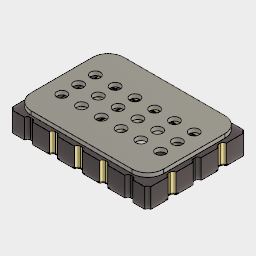
mics-6814_three_gas_sensor.7066ebe4-298e-4c48-8aa3-1ca8056fe42b (Autodesk Fusion 360 design; units mm, degrees)
Autodesk Fusion 360 part; units mm, degrees
sketch "Sketch1" plane through (0, 0, 0) normal (0, 0, 1) x (1, 0, 0) in component "body"
  line L0 (-3.5, 2.5) -> (3.5, 2.5)
  line L1 (3.5, 2.5) -> (3.5, -2.5)
  line L2 (3.5, -2.5) -> (-3.5, -2.5)
  line L3 (-3.5, -2.5) -> (-3.5, 2.5)
  arc A0 (3.35, 2.5) -> (3.5, 2.35) centre (3.5, 2.5) ccw
  arc A1 (3.5, -2.35) -> (3.35, -2.5) centre (3.5, -2.5) ccw
  arc A2 (-3.5, 2.35) -> (-3.35, 2.5) centre (-3.5, 2.5) ccw
  arc A3 (-3.35, -2.5) -> (-3.5, -2.35) centre (-3.5, -2.5) ccw
  line L4 (-0.3, 2.5) -> (0.3, 2.5)
  line L5 (0.3, 2.5) -> (0.3, 1.5)
  line L6 (0.3, 1.5) -> (-0.3, 1.5)
  line L7 (-0.3, 1.5) -> (-0.3, 2.5)
  line L8 (-0.05, 2.35) -> (0.05, 2.35)
  arc A4 (0.05, 2.35) -> (0.2, 2.5) centre (0.05, 2.5) ccw
  arc A5 (-0.2, 2.5) -> (-0.05, 2.35) centre (-0.05, 2.5) ccw
  arc A6 (-2.74, 2.5) -> (-2.59, 2.35) centre (-2.59, 2.5) ccw
  line L9 (-2.59, 2.35) -> (-2.49, 2.35)
  arc A7 (-2.49, 2.35) -> (-2.34, 2.5) centre (-2.49, 2.5) ccw
  arc A8 (-1.47, 2.5) -> (-1.32, 2.35) centre (-1.32, 2.5) ccw
  line L10 (-1.32, 2.35) -> (-1.22, 2.35)
  arc A9 (-1.22, 2.35) -> (-1.07, 2.5) centre (-1.22, 2.5) ccw
  arc A10 (1.07, 2.5) -> (1.22, 2.35) centre (1.22, 2.5) ccw
  line L11 (1.22, 2.35) -> (1.32, 2.35)
  arc A11 (1.32, 2.35) -> (1.47, 2.5) centre (1.32, 2.5) ccw
  arc A12 (2.34, 2.5) -> (2.49, 2.35) centre (2.49, 2.5) ccw
  line L12 (2.49, 2.35) -> (2.59, 2.35)
  arc A13 (2.59, 2.35) -> (2.74, 2.5) centre (2.59, 2.5) ccw
  line L13 (-3.5, 0) -> (3.5, 0) construction
  line L14 (3.35, 0.05) -> (3.35, -0.05)
  arc A14 (3.35, -0.05) -> (3.5, -0.2) centre (3.5, -0.05) ccw
  arc A15 (3.5, 0.2) -> (3.35, 0.05) centre (3.5, 0.05) ccw
  line L15 (-0.05, -2.35) -> (0.05, -2.35)
  arc A16 (0.2, -2.5) -> (0.05, -2.35) centre (0.05, -2.5) ccw
  arc A17 (-0.05, -2.35) -> (-0.2, -2.5) centre (-0.05, -2.5) ccw
  arc A18 (-2.59, -2.35) -> (-2.74, -2.5) centre (-2.59, -2.5) ccw
  line L16 (-2.59, -2.35) -> (-2.49, -2.35)
  arc A19 (-2.34, -2.5) -> (-2.49, -2.35) centre (-2.49, -2.5) ccw
  arc A20 (-1.32, -2.35) -> (-1.47, -2.5) centre (-1.32, -2.5) ccw
  line L17 (-1.32, -2.35) -> (-1.22, -2.35)
  arc A21 (-1.07, -2.5) -> (-1.22, -2.35) centre (-1.22, -2.5) ccw
  arc A22 (1.22, -2.35) -> (1.07, -2.5) centre (1.22, -2.5) ccw
  line L18 (1.22, -2.35) -> (1.32, -2.35)
  arc A23 (1.47, -2.5) -> (1.32, -2.35) centre (1.32, -2.5) ccw
  arc A24 (2.49, -2.35) -> (2.34, -2.5) centre (2.49, -2.5) ccw
  line L19 (2.49, -2.35) -> (2.59, -2.35)
  arc A25 (2.74, -2.5) -> (2.59, -2.35) centre (2.59, -2.5) ccw
  arc A26 (3.5, -1.07) -> (3.35, -1.22) centre (3.5, -1.22) ccw
  line L20 (3.35, -1.22) -> (3.35, -1.32)
  arc A27 (3.35, -1.32) -> (3.5, -1.47) centre (3.5, -1.32) ccw
  arc A28 (3.5, 1.47) -> (3.35, 1.32) centre (3.5, 1.32) ccw
  line L21 (3.35, 1.32) -> (3.35, 1.22)
  arc A29 (3.35, 1.22) -> (3.5, 1.07) centre (3.5, 1.22) ccw
  line L22 (-3.35, 0.05) -> (-3.35, -0.05)
  arc A30 (-3.5, -0.2) -> (-3.35, -0.05) centre (-3.5, -0.05) ccw
  arc A31 (-3.35, 0.05) -> (-3.5, 0.2) centre (-3.5, 0.05) ccw
  arc A32 (-3.35, -1.22) -> (-3.5, -1.07) centre (-3.5, -1.22) ccw
  line L23 (-3.35, -1.22) -> (-3.35, -1.32)
  arc A33 (-3.5, -1.47) -> (-3.35, -1.32) centre (-3.5, -1.32) ccw
  arc A34 (-3.35, 1.32) -> (-3.5, 1.47) centre (-3.5, 1.32) ccw
  line L24 (-3.35, 1.32) -> (-3.35, 1.22)
  arc A35 (-3.5, 1.07) -> (-3.35, 1.22) centre (-3.5, 1.22) ccw
  line L25 (-0.97, 2.5) -> (-0.97, 1.5)
  line L26 (-0.97, 1.5) -> (-1.57, 1.5)
  line L27 (-1.57, 1.5) -> (-1.57, 2.5)
  line L28 (1.57, 2.5) -> (1.57, 1.5)
  line L29 (1.57, 1.5) -> (0.97, 1.5)
  line L30 (0.97, 1.5) -> (0.97, 2.5)
  line L31 (-0.3, -2.5) -> (-0.3, -1.5)
  line L32 (-0.3, -1.5) -> (0.3, -1.5)
  line L33 (0.3, -1.5) -> (0.3, -2.5)
  line L34 (-1.57, -2.5) -> (-1.57, -1.5)
  line L35 (-1.57, -1.5) -> (-0.97, -1.5)
  line L36 (-0.97, -1.5) -> (-0.97, -2.5)
  line L37 (0.97, -2.5) -> (0.97, -1.5)
  line L38 (0.97, -1.5) -> (1.57, -1.5)
  line L39 (1.57, -1.5) -> (1.57, -2.5)
  line L40 (3.5, -0.97) -> (2.5, -0.97)
  line L41 (2.5, -0.97) -> (2.5, -1.57)
  line L42 (2.5, -1.57) -> (3.5, -1.57)
  line L43 (3.5, 1.57) -> (2.5, 1.57)
  line L44 (2.5, 1.57) -> (2.5, 0.97)
  line L45 (2.5, 0.97) -> (3.5, 0.97)
  line L46 (-3.5, 1.57) -> (-2.5, 1.57)
  line L47 (-2.5, 1.57) -> (-2.5, 0.97)
  line L48 (-2.5, 0.97) -> (-3.5, 0.97)
  line L49 (-3.5, -0.97) -> (-2.5, -0.97)
  line L50 (-2.5, -0.97) -> (-2.5, -1.57)
  line L51 (-2.5, -1.57) -> (-3.5, -1.57)
  circle A36 centre (1.25, 0.97) radius 0.2
  dimension "d1" = 5
  dimension "d2" = 7
  dimension "d3" = 0.3
  dimension "d4" = 0.3
  dimension "d5" = 0.3
  dimension "d6" = 0.3
  dimension "d8" = 0.6
  dimension "d9" = 1
  dimension "d10" = 0.15
  dimension "d11" = 0.15
  dimension "d12" = 0.15
  dimension "d13" = 0.4
  dimension "d16" = 1.27
  dimension "d17" = 0
  dimension "d18" = 0.15
  dimension "d19" = 0.15
  dimension "d20" = 0.15
  dimension "d21" = 0.4
  dimension "d27" = 0.15
  dimension "d28" = 0.15
  dimension "d29" = 0.4
  dimension "d32" = 1.27
  dimension "d33" = 0
  dimension "d34" = 0.15
  dimension "d37" = 0
  dimension "d38" = 1.27
  dimension "d39" = 0.15
  dimension "d40" = 0.15
  dimension "d41" = 0.15
  dimension "d42" = 0.4
  dimension "d45" = 0
  dimension "d46" = 1.27
  dimension "d49" = 1.27
  dimension "d50" = 0
  dimension "d51" = 1
  dimension "d52" = 0.6
  dimension "d55" = 1.27
  dimension "d56" = 0
  dimension "d57" = 1
  dimension "d58" = 0.6
  dimension "d59" = 1
  dimension "d60" = 0.6
  dimension "d61" = 1
  dimension "d62" = 0.6
  dimension "d63" = 1
  dimension "d64" = 0.6
  dimension "d65" = 0.4
  dimension "d67" = 1.25
  dimension "d92" = 0.97
  constraint horizontal L0
  constraint vertical L1
  constraint horizontal L2
  constraint vertical L3
  constraint coincident L1
  constraint coincident L0
  constraint coincident L2
  constraint coincident L3
  constraint midpoint L3
  constraint midpoint L0
  constraint horizontal L4
  constraint vertical L5
  constraint horizontal L6
  constraint vertical L7
  constraint midpoint L6
  constraint horizontal L8
  constraint coincident L4
  constraint tangent L8 A4
  constraint tangent L8 A5
  constraint midpoint L8
  constraint midpoint L1
  constraint tangent L14 A14
  constraint tangent L14 A15
  constraint vertical L14
  constraint tangent L15 A16
  constraint tangent L15 A17
  constraint horizontal L15
  constraint midpoint L15
  constraint tangent L22 A30
  constraint tangent L22 A31
  constraint vertical L22
  constraint midpoint L22
  constraint horizontal L32
  constraint vertical L31
  constraint vertical L33
  constraint midpoint L32
  constraint vertical L41
  constraint horizontal L40
  constraint horizontal L42
  constraint midpoint L41
  constraint midpoint L20
  constraint midpoint L44
  constraint midpoint L21
  constraint vertical L44
  constraint horizontal L43
  constraint horizontal L45
  constraint midpoint L47
  constraint midpoint L24
  constraint horizontal L46
  constraint horizontal L48
  constraint vertical L47
  constraint midpoint L50
  constraint midpoint L23
  constraint horizontal L49
  constraint horizontal L51
  constraint vertical L50
  constraint midpoint L14
  measures "d2" distance of L1 L3
  measures "d3" diameter of A2
  measures "d4" diameter of A3
  measures "d5" diameter of A1
  measures "d6" diameter of A0
  measures "d10" distance of L0 L8
  measures "d11" radius of A4
  measures "d12" radius of A5
  measures "d18" distance of L1 L14
  measures "d19" radius of A14
  measures "d20" radius of A15
  measures "d27" radius of A16
  measures "d28" radius of A17
  measures "d34" distance of L2
  measures "d39" distance of L3 L22
  measures "d40" radius of A31
  measures "d41" radius of A30
  measures "d51" distance of L2 L32
  measures "d52" distance of L31 L33
  measures "d57" distance of L1 L41
  measures "d58" distance of L40 L42
  measures "d59" distance of L1 L44
  measures "d60" distance of L43 L45
  measures "d61" distance of L3 L47
  measures "d62" distance of L46 L48
  measures "d63" distance of L3 L50
  measures "d64" distance of L49 L51
  measures "d65" diameter of A36
extrude "Extrude1" add sketch "Sketch1" along normal blind 1 contours L0 L1 L2 L3 A0 A1 A2 A3 L5 L6 L7 A6 L9 A7 A12 L12 A13 L14 A14 A15 A18 L16 A19 A24 L19 A25 L22 A30 A31 L25 L26 L27 L28 L29 L30 L31 L32 L33 L34 L35 L36 L37 L38 L39 L40 L41 L42 L43 L44 L45 L46 L47 L48 L49 L50 L51 | L3 A34 L24 A35 L46 L47 L48 | L0 A8 L10 A9 L25 L26 L27 | L0 L4 L5 L6 L7 L8 A4 A5 | L3 A32 L23 A33 L49 L50 L51 | L0 A10 L11 A11 L28 L29 L30 | L2 A20 L17 A21 L34 L35 L36 | L1 A28 L21 A29 L43 L44 L45 | L2 L15 A16 A17 L31 L32 L33 | L2 A22 L18 A23 L37 L38 L39 | L1 A26 L20 A27 L40 L41 L42 | A36 makes body 1 in component "body"
extrude "Extrude2" add sketch "Sketch1" along normal blind 0.05 separate body contours L3 A34 L24 A35 L46 L47 L48 | L0 A8 L10 A9 L25 L26 L27 | L0 L4 L5 L6 L7 L8 A4 A5 | L3 A32 L23 A33 L49 L50 L51 | L0 A10 L11 A11 L28 L29 L30 | L2 A20 L17 A21 L34 L35 L36 | L1 A28 L21 A29 L43 L44 L45 | L2 L15 A16 A17 L31 L32 L33 | L2 A22 L18 A23 L37 L38 L39 | L1 A26 L20 A27 L40 L41 L42 | A36 makes body 2 at (-0.0167, -1.7833, 0) makes body 3 at (-1.2533, 1.7833, 0) makes body 4 at (2.7833, -1.2867, 0) makes body 5 at (0.0167, 1.7833, 0) makes body 6 at (-1.2867, -1.7833, 0) makes body 7 at (1.2867, -1.7833, 0) makes body 8 at (-2.7833, 1.2533, 0) makes body 9 at (2.7833, 1.2867, 0) makes body 10 at (1.2867, 1.7833, 0) makes body 11 at (-2.7833, -1.2533, 0) makes body 12 at (1.4078, 0.9411, 0) in component "body"
combine "Combine1" operation cut target body 1 tool bodies 7 2 6 11 8 3 5 10 12 4 9 keep tools in component "body"
sketch "Sketch1 (2)" plane through (0, 0, 1) normal (0, 0, 1) x (-1, 0, 0) in component "lid"
  line L0 (3.35, -0.05) -> (3.35, 0.05)
  arc A0 (3.5, 0.2) -> (3.35, 0.05) centre (3.5, 0.05) ccw
  line L1 (3.5, 0.2) -> (3.5, 1.07)
  arc A1 (3.35, 1.22) -> (3.5, 1.07) centre (3.5, 1.22) ccw
  line L2 (3.35, 1.22) -> (3.35, 1.32)
  arc A2 (3.5, 1.47) -> (3.35, 1.32) centre (3.5, 1.32) ccw
  line L3 (3.5, 1.47) -> (3.5, 2.35)
  arc A3 (3.35, 2.5) -> (3.5, 2.35) centre (3.5, 2.5) ccw
  line L4 (3.35, 2.5) -> (2.74, 2.5)
  arc A4 (2.59, 2.35) -> (2.74, 2.5) centre (2.59, 2.5) ccw
  line L5 (2.59, 2.35) -> (2.49, 2.35)
  arc A5 (2.34, 2.5) -> (2.49, 2.35) centre (2.49, 2.5) ccw
  line L6 (2.34, 2.5) -> (1.47, 2.5)
  arc A6 (1.32, 2.35) -> (1.47, 2.5) centre (1.32, 2.5) ccw
  line L7 (1.32, 2.35) -> (1.22, 2.35)
  arc A7 (1.07, 2.5) -> (1.22, 2.35) centre (1.22, 2.5) ccw
  line L8 (1.07, 2.5) -> (0.2, 2.5)
  arc A8 (0.05, 2.35) -> (0.2, 2.5) centre (0.05, 2.5) ccw
  line L9 (0.05, 2.35) -> (-0.05, 2.35)
  arc A9 (-0.2, 2.5) -> (-0.05, 2.35) centre (-0.05, 2.5) ccw
  line L10 (-0.2, 2.5) -> (-1.07, 2.5)
  arc A10 (-1.22, 2.35) -> (-1.07, 2.5) centre (-1.22, 2.5) ccw
  line L11 (-1.22, 2.35) -> (-1.32, 2.35)
  arc A11 (-1.47, 2.5) -> (-1.32, 2.35) centre (-1.32, 2.5) ccw
  line L12 (-1.47, 2.5) -> (-2.34, 2.5)
  arc A12 (-2.49, 2.35) -> (-2.34, 2.5) centre (-2.49, 2.5) ccw
  line L13 (-2.49, 2.35) -> (-2.59, 2.35)
  arc A13 (-2.74, 2.5) -> (-2.59, 2.35) centre (-2.59, 2.5) ccw
  line L14 (-2.74, 2.5) -> (-3.35, 2.5)
  arc A14 (-3.5, 2.35) -> (-3.35, 2.5) centre (-3.5, 2.5) ccw
  line L15 (-3.5, 2.35) -> (-3.5, 1.47)
  arc A15 (-3.35, 1.32) -> (-3.5, 1.47) centre (-3.5, 1.32) ccw
  line L16 (-3.35, 1.32) -> (-3.35, 1.22)
  arc A16 (-3.5, 1.07) -> (-3.35, 1.22) centre (-3.5, 1.22) ccw
  line L17 (-3.5, 1.07) -> (-3.5, 0.2)
  arc A17 (-3.35, 0.05) -> (-3.5, 0.2) centre (-3.5, 0.05) ccw
  line L18 (-3.35, 0.05) -> (-3.35, -0.05)
  arc A18 (-3.5, -0.2) -> (-3.35, -0.05) centre (-3.5, -0.05) ccw
  line L19 (-3.5, -0.2) -> (-3.5, -1.07)
  arc A19 (-3.35, -1.22) -> (-3.5, -1.07) centre (-3.5, -1.22) ccw
  line L20 (-3.35, -1.22) -> (-3.35, -1.32)
  arc A20 (-3.5, -1.47) -> (-3.35, -1.32) centre (-3.5, -1.32) ccw
  line L21 (-3.5, -1.47) -> (-3.5, -2.35)
  arc A21 (-3.35, -2.5) -> (-3.5, -2.35) centre (-3.5, -2.5) ccw
  line L22 (-3.35, -2.5) -> (-2.74, -2.5)
  arc A22 (-2.59, -2.35) -> (-2.74, -2.5) centre (-2.59, -2.5) ccw
  line L23 (-2.59, -2.35) -> (-2.49, -2.35)
  arc A23 (-2.34, -2.5) -> (-2.49, -2.35) centre (-2.49, -2.5) ccw
  line L24 (-2.34, -2.5) -> (-1.47, -2.5)
  arc A24 (-1.32, -2.35) -> (-1.47, -2.5) centre (-1.32, -2.5) ccw
  line L25 (-1.32, -2.35) -> (-1.22, -2.35)
  arc A25 (-1.07, -2.5) -> (-1.22, -2.35) centre (-1.22, -2.5) ccw
  line L26 (-1.07, -2.5) -> (-0.2, -2.5)
  arc A26 (-0.05, -2.35) -> (-0.2, -2.5) centre (-0.05, -2.5) ccw
  line L27 (-0.05, -2.35) -> (0.05, -2.35)
  arc A27 (0.2, -2.5) -> (0.05, -2.35) centre (0.05, -2.5) ccw
  line L28 (0.2, -2.5) -> (1.07, -2.5)
  arc A28 (1.22, -2.35) -> (1.07, -2.5) centre (1.22, -2.5) ccw
  line L29 (1.22, -2.35) -> (1.32, -2.35)
  arc A29 (1.47, -2.5) -> (1.32, -2.35) centre (1.32, -2.5) ccw
  line L30 (1.47, -2.5) -> (2.34, -2.5)
  arc A30 (2.49, -2.35) -> (2.34, -2.5) centre (2.49, -2.5) ccw
  line L31 (2.49, -2.35) -> (2.59, -2.35)
  arc A31 (2.74, -2.5) -> (2.59, -2.35) centre (2.59, -2.5) ccw
  line L32 (2.74, -2.5) -> (3.35, -2.5)
  arc A32 (3.5, -2.35) -> (3.35, -2.5) centre (3.5, -2.5) ccw
  line L33 (3.5, -2.35) -> (3.5, -1.47)
  arc A33 (3.35, -1.32) -> (3.5, -1.47) centre (3.5, -1.32) ccw
  line L34 (3.35, -1.32) -> (3.35, -1.22)
  arc A34 (3.5, -1.07) -> (3.35, -1.22) centre (3.5, -1.22) ccw
  line L35 (3.5, -1.07) -> (3.5, -0.2)
  arc A35 (3.35, -0.05) -> (3.5, -0.2) centre (3.5, -0.05) ccw
  line L36 (2.55, -2.35) -> (-2.55, -2.35)
  line L37 (-3.35, -1.55) -> (-3.35, 1.55)
  line L38 (-2.55, 2.35) -> (2.55, 2.35)
  line L39 (3.35, 1.55) -> (3.35, -1.55)
  arc A36 (2.55, -2.35) -> (3.35, -1.55) centre (2.55, -1.55) ccw
  arc A37 (3.35, 1.55) -> (2.55, 2.35) centre (2.55, 1.55) ccw
  arc A38 (-3.35, -1.55) -> (-2.55, -2.35) centre (-2.55, -1.55) ccw
  arc A39 (-2.55, 2.35) -> (-3.35, 1.55) centre (-2.55, 1.55) ccw
  circle A40 centre (2.5, 0) radius 0.25
  circle A41 centre (2.5, -0.85) radius 0.25
  circle A42 centre (1.5, -0.85) radius 0.25
  circle A43 centre (0.5, -0.85) radius 0.25
  circle A44 centre (-0.5, -0.85) radius 0.25
  circle A45 centre (-1.5, -0.85) radius 0.25
  circle A46 centre (-2.5, -0.85) radius 0.25
  circle A47 centre (1.5, 0) radius 0.25
  circle A48 centre (0.5, 0) radius 0.25
  circle A49 centre (-0.5, 0) radius 0.25
  circle A50 centre (-1.5, 0) radius 0.25
  circle A51 centre (-2.5, 0) radius 0.25
  circle A52 centre (2.5, 0.85) radius 0.25
  circle A53 centre (1.5, 0.85) radius 0.25
  circle A54 centre (0.5, 0.85) radius 0.25
  circle A55 centre (-0.5, 0.85) radius 0.25
  circle A56 centre (-1.5, 0.85) radius 0.25
  circle A57 centre (-2.5, 0.85) radius 0.25
  dimension "d72" = 4.7
  dimension "d73" = 6.7
  dimension "d74" = 0.8
  dimension "d75" = 0.5
  dimension "d76" = 2.5
  dimension "d79" = -5
  dimension "d80" = 0.85
  constraint horizontal L36
  constraint vertical L37
  constraint horizontal L38
  constraint vertical L39
  constraint midpoint L36
  constraint midpoint L37
  constraint tangent L36 A36
  constraint tangent L39 A36
  constraint tangent L38 A37
  constraint tangent L39 A37
  constraint equal A36 A37
  constraint tangent L36 A38
  constraint tangent L37 A38
  constraint equal A36 A38
  constraint tangent L37 A39
  constraint tangent L38 A39
  constraint equal A36 A39
  measures "d72" distance of L36 L38
  measures "d73" distance of L37 L39
  measures "d74" radius of A36
  measures "d75" diameter of A40
extrude "Extrude1'" add sketch "Sketch1 (2)" along normal blind 0.2 separate body contours L0 L2 L5 L7 L9 L11 L13 L16 L18 L20 L23 L25 L27 L29 L31 L34 L36 L37 L38 L39 A36 A37 A38 A39 makes body 13 in component "lid"
move_body "MoveBody1" bodies 13 to x (1, 0, 0) y (0, 1, 0) z (0, 0, 1) at (0, 0, 0.1) in component "lid"
sketch "Sketch1 (1)" plane through (0, 0, 1) normal (0, 0, 1) x (-1, 0, 0) in component "body"
  line L0 (3.35, -0.05) -> (3.35, 0.05)
  arc A0 (3.5, 0.2) -> (3.35, 0.05) centre (3.5, 0.05) ccw
  line L1 (3.5, 0.2) -> (3.5, 1.07)
  arc A1 (3.35, 1.22) -> (3.5, 1.07) centre (3.5, 1.22) ccw
  line L2 (3.35, 1.22) -> (3.35, 1.32)
  arc A2 (3.5, 1.47) -> (3.35, 1.32) centre (3.5, 1.32) ccw
  line L3 (3.5, 1.47) -> (3.5, 2.35)
  arc A3 (3.35, 2.5) -> (3.5, 2.35) centre (3.5, 2.5) ccw
  line L4 (3.35, 2.5) -> (2.74, 2.5)
  arc A4 (2.59, 2.35) -> (2.74, 2.5) centre (2.59, 2.5) ccw
  line L5 (2.59, 2.35) -> (2.49, 2.35)
  arc A5 (2.34, 2.5) -> (2.49, 2.35) centre (2.49, 2.5) ccw
  line L6 (2.34, 2.5) -> (1.47, 2.5)
  arc A6 (1.32, 2.35) -> (1.47, 2.5) centre (1.32, 2.5) ccw
  line L7 (1.32, 2.35) -> (1.22, 2.35)
  arc A7 (1.07, 2.5) -> (1.22, 2.35) centre (1.22, 2.5) ccw
  line L8 (1.07, 2.5) -> (0.2, 2.5)
  arc A8 (0.05, 2.35) -> (0.2, 2.5) centre (0.05, 2.5) ccw
  line L9 (0.05, 2.35) -> (-0.05, 2.35)
  arc A9 (-0.2, 2.5) -> (-0.05, 2.35) centre (-0.05, 2.5) ccw
  line L10 (-0.2, 2.5) -> (-1.07, 2.5)
  arc A10 (-1.22, 2.35) -> (-1.07, 2.5) centre (-1.22, 2.5) ccw
  line L11 (-1.22, 2.35) -> (-1.32, 2.35)
  arc A11 (-1.47, 2.5) -> (-1.32, 2.35) centre (-1.32, 2.5) ccw
  line L12 (-1.47, 2.5) -> (-2.34, 2.5)
  arc A12 (-2.49, 2.35) -> (-2.34, 2.5) centre (-2.49, 2.5) ccw
  line L13 (-2.49, 2.35) -> (-2.59, 2.35)
  arc A13 (-2.74, 2.5) -> (-2.59, 2.35) centre (-2.59, 2.5) ccw
  line L14 (-2.74, 2.5) -> (-3.35, 2.5)
  arc A14 (-3.5, 2.35) -> (-3.35, 2.5) centre (-3.5, 2.5) ccw
  line L15 (-3.5, 2.35) -> (-3.5, 1.47)
  arc A15 (-3.35, 1.32) -> (-3.5, 1.47) centre (-3.5, 1.32) ccw
  line L16 (-3.35, 1.32) -> (-3.35, 1.22)
  arc A16 (-3.5, 1.07) -> (-3.35, 1.22) centre (-3.5, 1.22) ccw
  line L17 (-3.5, 1.07) -> (-3.5, 0.2)
  arc A17 (-3.35, 0.05) -> (-3.5, 0.2) centre (-3.5, 0.05) ccw
  line L18 (-3.35, 0.05) -> (-3.35, -0.05)
  arc A18 (-3.5, -0.2) -> (-3.35, -0.05) centre (-3.5, -0.05) ccw
  line L19 (-3.5, -0.2) -> (-3.5, -1.07)
  arc A19 (-3.35, -1.22) -> (-3.5, -1.07) centre (-3.5, -1.22) ccw
  line L20 (-3.35, -1.22) -> (-3.35, -1.32)
  arc A20 (-3.5, -1.47) -> (-3.35, -1.32) centre (-3.5, -1.32) ccw
  line L21 (-3.5, -1.47) -> (-3.5, -2.35)
  arc A21 (-3.35, -2.5) -> (-3.5, -2.35) centre (-3.5, -2.5) ccw
  line L22 (-3.35, -2.5) -> (-2.74, -2.5)
  arc A22 (-2.59, -2.35) -> (-2.74, -2.5) centre (-2.59, -2.5) ccw
  line L23 (-2.59, -2.35) -> (-2.49, -2.35)
  arc A23 (-2.34, -2.5) -> (-2.49, -2.35) centre (-2.49, -2.5) ccw
  line L24 (-2.34, -2.5) -> (-1.47, -2.5)
  arc A24 (-1.32, -2.35) -> (-1.47, -2.5) centre (-1.32, -2.5) ccw
  line L25 (-1.32, -2.35) -> (-1.22, -2.35)
  arc A25 (-1.07, -2.5) -> (-1.22, -2.35) centre (-1.22, -2.5) ccw
  line L26 (-1.07, -2.5) -> (-0.2, -2.5)
  arc A26 (-0.05, -2.35) -> (-0.2, -2.5) centre (-0.05, -2.5) ccw
  line L27 (-0.05, -2.35) -> (0.05, -2.35)
  arc A27 (0.2, -2.5) -> (0.05, -2.35) centre (0.05, -2.5) ccw
  line L28 (0.2, -2.5) -> (1.07, -2.5)
  arc A28 (1.22, -2.35) -> (1.07, -2.5) centre (1.22, -2.5) ccw
  line L29 (1.22, -2.35) -> (1.32, -2.35)
  arc A29 (1.47, -2.5) -> (1.32, -2.35) centre (1.32, -2.5) ccw
  line L30 (1.47, -2.5) -> (2.34, -2.5)
  arc A30 (2.49, -2.35) -> (2.34, -2.5) centre (2.49, -2.5) ccw
  line L31 (2.49, -2.35) -> (2.59, -2.35)
  arc A31 (2.74, -2.5) -> (2.59, -2.35) centre (2.59, -2.5) ccw
  line L32 (2.74, -2.5) -> (3.35, -2.5)
  arc A32 (3.5, -2.35) -> (3.35, -2.5) centre (3.5, -2.5) ccw
  line L33 (3.5, -2.35) -> (3.5, -1.47)
  arc A33 (3.35, -1.32) -> (3.5, -1.47) centre (3.5, -1.32) ccw
  line L34 (3.35, -1.32) -> (3.35, -1.22)
  arc A34 (3.5, -1.07) -> (3.35, -1.22) centre (3.5, -1.22) ccw
  line L35 (3.5, -1.07) -> (3.5, -0.2)
  arc A35 (3.35, -0.05) -> (3.5, -0.2) centre (3.5, -0.05) ccw
  line L36 (2.575, -1.875) -> (-2.575, -1.875)
  line L37 (-2.875, -1.575) -> (-2.875, 1.575)
  line L38 (-2.575, 1.875) -> (2.575, 1.875)
  line L39 (2.875, 1.575) -> (2.875, -1.575)
  arc A36 (2.575, -1.875) -> (2.875, -1.575) centre (2.575, -1.575) ccw
  arc A37 (-2.875, -1.575) -> (-2.575, -1.875) centre (-2.575, -1.575) ccw
  arc A38 (-2.575, 1.875) -> (-2.875, 1.575) centre (-2.575, 1.575) ccw
  arc A39 (2.875, 1.575) -> (2.575, 1.875) centre (2.575, 1.575) ccw
  dimension "d83" = 3.75
  dimension "d84" = 5.75
  dimension "d85" = 0.3
  constraint horizontal L36
  constraint vertical L37
  constraint horizontal L38
  constraint vertical L39
  constraint midpoint L37
  constraint midpoint L38
  constraint tangent L36 A36
  constraint tangent L39 A36
  constraint tangent L36 A37
  constraint tangent L37 A37
  constraint equal A36 A37
  constraint tangent L37 A38
  constraint tangent L38 A38
  constraint equal A36 A38
  constraint tangent L38 A39
  constraint tangent L39 A39
  constraint equal A36 A39
  measures "d83" distance of L36 L38
  measures "d84" distance of L37 L39
  measures "d85" radius of A36
extrude "Extrude3" cut sketch "Sketch1 (1)" against normal blind 0.5 contours L36 L37 L38 L39 A36 A37 A38 A39 bodies 1 in component "body"
sketch "Sketch2" plane through (0, 0, 0.5) normal (0, 0, 1) x (-1, 0, 0) in component "body"
  arc A0 (2.575, -1.875) -> (2.875, -1.575) centre (2.575, -1.575) ccw
  line L0 (2.875, -1.575) -> (2.875, 1.575)
  arc A1 (2.875, 1.575) -> (2.575, 1.875) centre (2.575, 1.575) ccw
  line L1 (2.575, 1.875) -> (-2.575, 1.875)
  arc A2 (-2.575, 1.875) -> (-2.875, 1.575) centre (-2.575, 1.575) ccw
  line L2 (-2.875, 1.575) -> (-2.875, -1.575)
  arc A3 (-2.875, -1.575) -> (-2.575, -1.875) centre (-2.575, -1.575) ccw
  line L3 (-2.575, -1.875) -> (2.575, -1.875)
  line L4 (2.75, -1.25) -> (-2.75, -1.25)
  line L5 (-2.75, -1.25) -> (-2.75, 1.25)
  line L6 (-2.75, 1.25) -> (2.75, 1.25)
  line L7 (2.75, 1.25) -> (2.75, -1.25)
  dimension "d88" = 2.5
  dimension "d89" = 5.5
  constraint horizontal L4
  constraint vertical L5
  constraint horizontal L6
  constraint vertical L7
  constraint midpoint L7
  constraint midpoint L4
extrude "Extrude4" add sketch "Sketch2" along normal blind 0.3 bodies 1 in component "body"
sketch "Sketch2 (1)" plane through (0, 0, 0.8) normal (0, 0, 1) x (-1, 0, 0) in component "body"
  line L0 (-2.75, 1.25) -> (2.75, 1.25)
  line L1 (2.75, 1.25) -> (2.75, -1.25)
  line L2 (2.75, -1.25) -> (-2.75, -1.25)
  line L3 (-2.75, -1.25) -> (-2.75, 1.25)
  line L4 (-2.575, -1.875) -> (2.575, -1.875)
  arc A0 (2.575, -1.875) -> (2.875, -1.575) centre (2.575, -1.575) ccw
  line L5 (2.875, -1.575) -> (2.875, 1.575)
  arc A1 (2.875, 1.575) -> (2.575, 1.875) centre (2.575, 1.575) ccw
  line L6 (2.575, 1.875) -> (-2.575, 1.875)
  arc A2 (-2.575, 1.875) -> (-2.875, 1.575) centre (-2.575, 1.575) ccw
  line L7 (-2.875, 1.575) -> (-2.875, -1.575)
  arc A3 (-2.875, -1.575) -> (-2.575, -1.875) centre (-2.575, -1.575) ccw
  arc A4 (2.575, -1.875) -> (2.875, -1.575) centre (2.575, -1.575) ccw
  line L8 (2.875, 1.575) -> (2.875, -1.575)
  line L9 (2.575, -1.875) -> (-2.575, -1.875)
  line L10 (2.75, -1.25) -> (-2.75, -1.25)
  line L11 (-2.75, 1.25) -> (2.75, 1.25)
  arc A5 (2.875, 1.575) -> (2.575, 1.875) centre (2.575, 1.575) ccw
  line L12 (-2.575, 1.875) -> (2.575, 1.875)
  arc A6 (-2.575, 1.875) -> (-2.875, 1.575) centre (-2.575, 1.575) ccw
  line L13 (-2.875, -1.575) -> (-2.875, 1.575)
  arc A7 (-2.875, -1.575) -> (-2.575, -1.875) centre (-2.575, -1.575) ccw
  line L14 (1.375, -1.25) -> (1.375, -1.875)
  line L15 (0.825, -1.25) -> (0.825, -1.875)
  line L16 (0.325, -1.25) -> (0.325, -1.875)
  line L17 (-0.225, -1.25) -> (-0.225, -1.875)
  line L18 (-0.725, -1.25) -> (-0.725, -1.875)
  line L19 (-1.275, -1.25) -> (-1.275, -1.875)
  line L20 (-1.775, -1.25) -> (-1.775, -1.875)
  line L21 (-2.275, -1.25) -> (-2.275, -1.575)
  line L22 (-2.275, -1.575) -> (-2.875, -1.575)
  line L23 (2.375, 1.25) -> (2.375, 1.575)
  line L24 (2.375, 1.575) -> (2.875, 1.575)
  line L25 (1.875, 1.25) -> (1.875, 1.875)
  line L26 (1.375, 1.25) -> (1.375, 1.875)
  line L27 (0.825, 1.25) -> (0.825, 1.875)
  line L28 (0.325, 1.25) -> (0.325, 1.875)
  line L29 (-0.225, 1.25) -> (-0.225, 1.875)
  line L30 (-0.725, 1.25) -> (-0.725, 1.875)
  line L31 (-1.275, 1.25) -> (-1.275, 1.875)
  line L32 (-1.775, 1.25) -> (-1.775, 1.875)
  line L33 (-2.275, 1.25) -> (-2.275, 1.575)
  line L34 (-2.275, 1.575) -> (-2.875, 1.575)
  line L35 (1.875, -1.875) -> (1.875, -1.25)
  line L36 (2.75, -1.25) -> (2.875, -1.25)
  dimension "d95" = 0.55
  dimension "d96" = 0.5
  dimension "d97" = 0.55
  dimension "d98" = 0.5
  dimension "d99" = 0.55
  dimension "d100" = 0.5
  dimension "d101" = 0.5
  dimension "d102" = 1
  dimension "d103" = 0.5
  dimension "d104" = 0.5
  dimension "d105" = 0.55
  dimension "d106" = 0.5
  dimension "d107" = 0.55
  dimension "d108" = 0.5
  dimension "d109" = 0.55
  dimension "d110" = 0.5
  dimension "d111" = 0.5
  dimension "d112" = 1
  dimension "d113" = 0.5
  constraint coincident L10
  constraint coincident L9
  constraint vertical L14
  constraint vertical L15
  constraint vertical L16
  constraint vertical L17
  constraint vertical L18
  constraint vertical L19
  constraint vertical L20
  constraint horizontal L22
  constraint vertical L21
  constraint coincident L11
  constraint horizontal L24
  constraint vertical L23
  constraint coincident L12
  constraint horizontal L34
  constraint vertical L33
  constraint vertical L32
  constraint vertical L31
  constraint vertical L30
  constraint vertical L29
  constraint vertical L28
  constraint vertical L27
  constraint vertical L26
  constraint vertical L25
  constraint vertical L35
  constraint coincident L8
  constraint horizontal L36
  measures "d95" distance of L14 L15
  measures "d96" distance of L15 L16
  measures "d97" distance of L16 L17
  measures "d98" distance of L17 L18
  measures "d99" distance of L18 L19
  measures "d100" distance of L19 L20
  measures "d101" distance of L20 L21
  measures "d102" distance of L8 L25
  measures "d103" distance of L23 L25
  measures "d104" distance of L25 L26
  measures "d105" distance of L26 L27
  measures "d106" distance of L27 L28
  measures "d107" distance of L28 L29
  measures "d108" distance of L29 L30
  measures "d109" distance of L30 L31
  measures "d110" distance of L31 L32
  measures "d111" distance of L32 L33
  measures "d112" distance of L8 L35
  measures "d113" distance of L14 L35
extrude "Extrude5" add sketch "Sketch2 (1)" against normal blind 0.05 separate body contours L0 L6 A2 L11 L12 A6 L32 L33 L34 | L2 L4 A3 L9 L10 A7 L20 L21 L22 | L0 L6 L11 L12 L30 L31 | L2 L4 L9 L10 L18 L19 | L0 L6 L11 L12 L28 L29 | L2 L4 L9 L10 L16 L17 | L0 L6 L11 L12 L26 L27 | L2 L4 L9 L10 L14 L15 | L0 A1 L6 L11 A5 L12 L23 L24 L25 | L2 L4 A0 L5 A4 L8 L9 L10 L35 L36 makes body 14 at (0.0417, -1.6667, 0.8) makes body 15 at (1.0917, 1.4583, 0.8) makes body 16 at (-2.4417, 1.4583, 0.8) makes body 17 at (1.9417, 1.5667, 0.8) makes body 18 at (-1.1917, -1.4583, 0.8) makes body 19 at (0.9083, -1.4583, 0.8) makes body 20 at (0.0417, 1.4583, 0.8) makes body 21 at (-1.1917, 1.6667, 0.8) makes body 22 at (1.9417, -1.5667, 0.8) makes body 23 at (-2.0417, -1.5667, 0.8) in component "body"
combine "Combine3" operation cut target body 1 tool bodies 16 21 20 15 17 22 19 14 18 23 keep tools in component "body"
sketch "Sketch1 (3)" plane through (0, 0, 0.5) normal (0, 0, 1) x (-1, 0, 0) in component "Component"
  line L0 (-2.75, 1.25) -> (-2.75, -1.25)
  line L1 (-2.75, -1.25) -> (2.75, -1.25)
  line L2 (2.75, -1.25) -> (2.75, 1.25)
  line L3 (2.75, 1.25) -> (-2.75, 1.25)
  line L4 (0.875, -1) -> (-0.875, -1)
  line L5 (-0.875, -1) -> (-0.875, 1)
  line L6 (-0.875, 1) -> (0.875, 1)
  line L7 (0.875, 1) -> (0.875, -1)
  dimension "d116" = 2
  dimension "d117" = 1.75
  constraint horizontal L4
  constraint vertical L5
  constraint horizontal L6
  constraint vertical L7
  constraint midpoint L5
  constraint midpoint L4
  measures "d117" distance of L5 L7
extrude "Extrude1''" add sketch "Sketch1 (3)" along normal blind 0.25 separate body contours L4 L5 L6 L7 makes body 24 in component "Component"
component "body" placed x (1, 0, 0) y (0, 1, 0) z (0, 0, 1) at (0, 0, 0)
component "lid" placed x (1, 0, 0) y (0, 1, 0) z (0, 0, 1) at (0, 0, 0)
component "Component" placed x (1, 0, 0) y (0, 1, 0) z (0, 0, 1) at (0, 0, 0.05)
component "Component" placed x (1, 0, 0) y (0, 1, 0) z (0, 0, 1) at (-1.8, 0, 0.05)
component "Component" placed x (1, 0, 0) y (0, 1, 0) z (0, 0, 1) at (1.8, 0, 0.05)
equation "d3 = ( 0.15 * 2 ) * 1 mm"
equation "d12 = d11"
equation "d18 = d10"
equation "d19 = d11"
equation "d20 = d11"
equation "d21 = d13"
equation "d27 = d11"
equation "d28 = d11"
equation "d29 = d13"
equation "d34 = d10"
equation "d39 = d10"
equation "d40 = d11"
equation "d41 = d11"
equation "d42 = d13"
equation "d51 = d9"
equation "d52 = d8"
equation "d57 = d9"
equation "d58 = d8"
equation "d59 = d9"
equation "d60 = d8"
equation "d61 = d9"
equation "d62 = d8"
equation "d63 = d9"
equation "d64 = d8"
equation "d72 = 5 mm - 0.3 mm"
equation "d73 = 7 mm - 0.3 mm"
